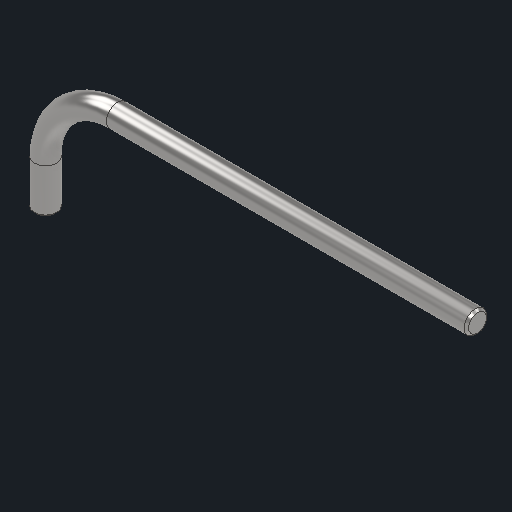
# Autodesk Inventor part: Lever
Saved by Autodesk Inventor 2025.4 (Build 294407000, 407)
## iProperties
Created: 2026-05-27
Part Number: Lever
Material: Stainless Steel
Document SubType Name: Modeling
Designer: VuQuan
Density: 8 g/cm^3
Appearance: Semi-Polished
Author: VuQuan
Autodesk Inventor part; units mm, degrees
ref_plane "YZ Plane" through (0, 0, 0) normal (1, 0, 0) x (0, 1, 0)
ref_plane "XZ Plane" through (0, 0, 0) normal (0, 1, 0) x (-1, 0, 0)
ref_plane "XY Plane" through (0, 0, 0) normal (0, 0, 1) x (1, 0, 0)
sketch "Sketch1" plane through (0, 0, 0) normal (0, 0, 1) x (1, 0, 0)
  line L0 (0, 0) -> (0, 10)
  arc A0 (16, 26) -> (0, 10) centre (16, 10) ccw
  line L1 (16, 26) -> (96, 26)
  dimension "d0" = 26
  dimension "d1" = 96
  dimension "d2" = 16
  constraints: 4 end point, 2 point on circle, 2 tangent, 1 centre point, 1 perpendicular, 1 vertical
  measures "d0" distance from line of L0.start L1
  measures "d1" distance from line of L1.end L0
  measures "d2" radius of A0
sketch "Sketch2" plane through (0, 0, 0) normal (0, 1, 0) x (-1, 0, 0)
  circle A0 centre (0, 0) radius 2.5
  dimension "d3" = 5
  constraints: 1 centre point, 1 coincident
  measures "d3" diameter of A0
sweep "Sweep1" add profiles "Sketch2" path "Sketch1"
chamfer "Chamfer1" distance 0.5 angle 45 4 edges at (2.5, 0, 0) (2.5, 10, 0) (16, 23.5, 0) (96, 23.5, 0)
body "Solid1"
